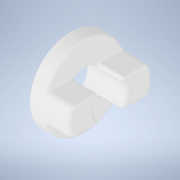
# Autodesk Inventor part: LED Washer
Saved by Autodesk Inventor 2020 (Build 240168000, 168)
## iProperties
Created: 2020-02-14
Part Number: LED Washer
Material: ABS Plastic
Document SubType Name: Modeling
Designer: Ishaan
Density: 1.06 g/cm^3
Appearance: Smooth - White
Author: Ishaan
Autodesk Inventor part; units mm, degrees
ref_plane "YZ Plane" through (0, 0, 0) normal (1, 0, 0) x (0, 1, 0)
ref_plane "XZ Plane" through (0, 0, 0) normal (0, 1, 0) x (-1, 0, 0)
ref_plane "XY Plane" through (0, 0, 0) normal (0, 0, 1) x (1, 0, 0)
sketch "Sketch1" plane through (0, 0, 0) normal (1, 0, 0) x (0, 1, 0)
  circle A0 centre (0, 0) radius 4
  line L0 (-1.375, -4) -> (1.375, -4)
  line L1 (1.375, -4) -> (1.375, 4)
  line L2 (1.375, 4) -> (-1.375, 4)
  line L3 (-1.375, 4) -> (-1.375, -4)
  line L4 (-1.375, -4) -> (1.375, 4) construction
  line L5 (1.375, -4) -> (-1.375, 4) construction
  point P0 (-1.375, 3.7562)
  point P1 (-1.375, -3.7562)
  point P2 (1.375, -3.7562)
  point P3 (1.375, 3.7562)
  dimension "d0" = 8
  dimension "d1" = 2.75
  constraints: 12 end point, 2 midpoint, 2 parallel, 1 centre point, 1 coincident, 1 horizontal, 1 perpendicular, 1 tangent
  measures "d0" diameter of A0
  measures "d1" distance of L2.end L1.end
extrude "Extrusion1" add sketch "Sketch1" against normal blind 1.5 contours A0 L1 | L1 A0 L3 | L3 A0
extrude "Extrusion2" add sketch "Sketch1" along normal blind 2.5 contours L1 A0 L3
sketch "Sketch2" plane through (-1.5, 0, 0) normal (-1, 0, 0) x (0, 0, 1)
  circle A0 centre (0, 0) radius 4 projected
  constraints: 1 coincident
hole "Hole1" at (-1.5, 0, 0) direction (1, 0, 0) diameter 3.2 end through all
fillet "Fillet1" radius 0.25 4 edges at (1.25, 1.375, 0.8182) (1.25, -1.375, 0.8182) (1.25, 1.375, -0.8182) (1.25, -1.375, -0.8182)
fillet "Fillet2" radius 0.5 4 edges at (1.25, 1.375, 3.7562) (1.25, -1.375, 3.7562) (1.25, 1.375, -3.7562) (1.25, -1.375, -3.7562)
fillet "Fillet3" radius 0.25 12 edges at (0, 1.2703, -3.695) (0, 1.2357, -1.2445) (0, 1.375, -2.4287) (0, 1.2357, 1.2445) (0, 1.2703, 3.695) (0, 1.375, 2.4287) (0, -1.2703, 3.695) (0, -1.2357, 1.2445) (0, -1.375, 2.4287) (0, -1.375, -2.4287) (0, -1.2357, -1.2445) (0, -1.2703, -3.695)
fillet "Fillet4" radius 0.25 26 edges at (2.5, 1.2703, 3.695) (2.5, 0, 4) (2.5, -1.2703, 3.695) (2.5, -1.375, 2.4287) (2.5, -1.2357, 1.2445) (2.5, -0.5137, 1.5153) (2.5, 0.5137, 1.5153) (2.5, 1.2357, 1.2445) (2.5, 1.375, 2.4287) (2.5, 1.2357, -1.2445) (2.5, 0, -1.6) (2.5, -1.2357, -1.2445) (2.5, -1.375, -2.4287) (2.5, -1.2703, -3.695) (2.5, 0, -4) (2.5, 1.2703, -3.695) (2.5, 1.375, -2.4287) (-1.5, -4, 0) (0.081, 1.2713, 3.7926) (0.081, 1.2713, -3.7926) (0, 3.3364, -2.2064) (0, 3.3364, 2.2064) (0.081, -1.2713, -3.7926) (0.081, -1.2713, 3.7926) (0, -4, 0) (-1.5, 0, -1.6)
fillet "Fillet5" radius 0.125 6 edges at (0.0862, 1.1039, -1.1582) (0.0862, 1.1039, 1.1582) (0, 1.6, 0) (0.0862, -1.1039, 1.1582) (0.0862, -1.1039, -1.1582) (0, -1.6, 0)
body "Solid1"
